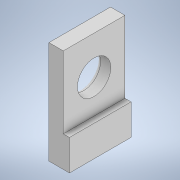
# Autodesk Inventor part: Bracket_Support
Saved by Autodesk Inventor 2022 (Build 260153000, 153)
## iProperties
Created: 2022-01-22
Part Number: Bracket_Support
Material: Generic
Document SubType Name: Modeling
Designer: Mlees
Density: 1 g/cm^3
Appearance: Default
Author: Mlees
Autodesk Inventor part; units mm, degrees
ref_plane "YZ Plane" through (0, 0, 0) normal (1, 0, 0) x (0, 1, 0)
ref_plane "XZ Plane" through (0, 0, 0) normal (0, 1, 0) x (-1, 0, 0)
ref_plane "XY Plane" through (0, 0, 0) normal (0, 0, 1) x (1, 0, 0)
sketch "Sketch1" plane through (0, 0, 0) normal (0, 1, 0) x (-1, 0, 0)
  line L0 (0, 0) -> (10, 0)
  line L1 (10, 0) -> (10, -30)
  line L2 (10, -30) -> (0, -30)
  line L3 (0, -30) -> (0, 0)
  dimension "d0" = 10
  dimension "d1" = 30
  constraints: 8 end point, 2 parallel, 1 horizontal, 1 perpendicular
  measures "d0" distance of L1.end L2.end
  measures "d1" distance of L0.end L1.end
extrude "Extrusion1" add sketch "Sketch1" along normal blind 50
sketch "Sketch2" plane through (0, 0, 0) normal (0, -1, 0) x (1, 0, 0)
  line L0 (0, 0) -> (0, -30) projected
  circle A0 centre (-5, -5) radius 1.5
  circle A1 centre (-5, -25) radius 1.5
  dimension "d7" = 3
  constraints: 2 centre point
  measures "d7" diameter of A0
extrude "Extrusion2" cut sketch "Sketch2" against normal blind 8
sketch "Sketch3" plane through (0, 0, 0) normal (1, 0, 0) x (0, 0, -1)
  line L0 (30, 0) -> (0, 0) projected
  circle A0 centre (15, 31.418) radius 8.125
  dimension "d11" = 16.25
  constraints: 1 centre point
  measures "d11" diameter of A0
extrude "Extrusion3" cut sketch "Sketch3" against normal up to surface (10 mm away)
fillet "Fillet1" radius 2 2 edges at (0, 31.418, -6.875) (-10, 31.418, -6.875)
sketch "Sketch5" plane through (0, 0, 0) normal (1, 0, 0) x (0, 0, -1)
  line L0 (30, 50) -> (0, 50) projected
  line L1 (30, 0) -> (30, 50) projected
  line L2 (0, 50) -> (30, 50)
  line L3 (30, 50) -> (30, 15)
  line L4 (30, 15) -> (0, 15)
  line L5 (0, 15) -> (0, 50)
  point P0 (0, 0)
  dimension "d15" = 35
  constraints: 8 end point, 2 parallel, 1 horizontal, 1 perpendicular, 1 point on line
  measures "d15" distance of L2.end L3.end
extrude "Extrusion4" cut sketch "Sketch5" against normal blind 3
body "Solid1"
